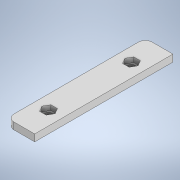
# Autodesk Inventor part: Rubberplate
Saved by Autodesk Inventor 2020.2 (Build 242310000, 310)
## iProperties
Created: 2021-06-22
Part Number: Rubberplate
Material: Generic
Document SubType Name: Modeling
Designer: JK
Density: 1 g/cm^3
Appearance: Default
Author: JK
Autodesk Inventor part; units mm, degrees
ref_plane "YZ Plane" through (0, 0, 0) normal (1, 0, 0) x (0, 1, 0)
ref_plane "XZ Plane" through (0, 0, 0) normal (0, 1, 0) x (-1, 0, 0)
ref_plane "XY Plane" through (0, 0, 0) normal (0, 0, 1) x (1, 0, 0)
sketch "Sketch1" plane through (0, 0, 0) normal (0, 1, 0) x (-1, 0, 0)
  line L0 (-10, 50) -> (10, 50)
  line L1 (10, 50) -> (10, -50)
  line L2 (10, -50) -> (-10, -50)
  line L3 (-10, -50) -> (-10, 50)
  line L4 (-10, 50) -> (10, -50) construction
  line L5 (10, 50) -> (-10, -50) construction
  circle A0 centre (0, 30) radius 2.75
  circle A1 centre (0, -30) radius 2.75
  point P0 (0, 0)
  dimension "d0" = 20
  dimension "d1" = 100
  dimension "d2" = 5.5
  dimension "d3" = 20
  dimension "d4" = 20
  constraints: 12 end point, 2 centre point, 2 midpoint, 2 parallel, 1 equal radius, 1 horizontal, 1 perpendicular
  measures "d0" distance between parallel lines of L1 L3
  measures "d1" distance of L0.end L1.end
  measures "d2" diameter of A0
  measures "d3" distance from line of L0 A0.centre
  measures "d4" distance from line of L2 A1.centre
extrude "Extrusion1" add sketch "Sketch1" along normal blind 5
sketch "Sketch2" plane through (0, 5, 0) normal (0, 1, 0) x (1, 0, 0)
  circle A0 centre (0, -30) radius 2.75 projected
  circle A1 centre (0, -30) radius 4.1
  circle A2 centre (0, 30) radius 2.75 projected
  circle A3 centre (0, 30) radius 4.1
  line L0 (-4.7343, -30) -> (-2.3671, -25.9)
  line L1 (-2.3671, -25.9) -> (2.3671, -25.9)
  line L2 (2.3671, -25.9) -> (4.7343, -30)
  line L3 (4.7343, -30) -> (2.3671, -34.1)
  line L4 (2.3671, -34.1) -> (-2.3671, -34.1)
  line L5 (-2.3671, -34.1) -> (-4.7343, -30)
  line L6 (-4.7343, 30) -> (-2.3671, 34.1)
  line L7 (-2.3671, 34.1) -> (2.3671, 34.1)
  line L8 (2.3671, 34.1) -> (4.7343, 30)
  line L9 (4.7343, 30) -> (2.3671, 25.9)
  line L10 (2.3671, 25.9) -> (-2.3671, 25.9)
  line L11 (-2.3671, 25.9) -> (-4.7343, 30)
  point P0 (0, 0)
  dimension "d7" = 8.2
  constraints: 24 end point, 4 coincident, 2 centre point, 2 horizontal alignment, 2 tangent, 1 equal radius, 26 other
  measures "d7" diameter of A1
extrude "Extrusion2" cut sketch "Sketch2" against normal blind 3.5 contours A0 | A1 | A1 L2 L3 | A1 L1 L2 | L3 L4 A1 | A1 L0 L1 | L4 L5 A1 | A1 L5 L0 | A2 | A3 | A3 L8 L9 | A3 L7 L8 | L9 L10 A3 | A3 L6 L7 | L10 L11 A3 | A3 L11 L6
fillet "Fillet1" radius 5 2 edges at (-10, 2.5, 50) (-10, 2.5, -50)
body "Solid1"
